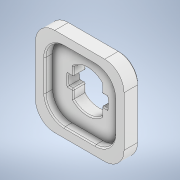
# Autodesk Inventor part: Capinsert_front
Saved by Autodesk Inventor 2021 (Build 250183000, 183)
## iProperties
Created: 2022-04-22
Part Number: Capinsert_front
Material: PPS-Kunststoff
Document SubType Name: Modeling
Designer: Timo
Density: 1.637 g/cm^3
Appearance: Glatt - Weiß
Mass: 2.02617 g
Surface Area: 14.372 cm^2
Volume: 1.23774 cm^3
Author: Timo
Autodesk Inventor part; units mm, degrees
ref_plane "YZ Plane" through (0, 0, 0) normal (1, 0, 0) x (0, 1, 0)
ref_plane "XZ Plane" through (0, 0, 0) normal (0, 1, 0) x (-1, 0, 0)
ref_plane "XY Plane" through (0, 0, 0) normal (0, 0, 1) x (1, 0, 0)
sketch "Skizze1" plane through (0, 0, 0) normal (0, 0, 1) x (1, 0, 0)
  line L0 (-11.45, -11.45) -> (11.45, -11.45)
  line L1 (11.45, -11.45) -> (11.45, 11.45)
  line L2 (11.45, 11.45) -> (-11.45, 11.45)
  line L3 (-11.45, 11.45) -> (-11.45, -11.45)
  line L4 (-11.45, -11.45) -> (11.45, 11.45) construction
  line L5 (11.45, -11.45) -> (-11.45, 11.45) construction
  point P0 (0, 0)
  dimension "d0" = 22.9
  constraints: 12 end point, 2 midpoint, 2 parallel, 2 perpendicular, 1 horizontal
  measures "d0" distance of L2.end L1.end
extrude "Extrusion1" add sketch "Skizze1" along normal blind 3.8
fillet "Rundung1" radius 5 4 edges at (11.45, 11.45, 1.9) (11.45, -11.45, 1.9) (-11.45, -11.45, 1.9) (-11.45, 11.45, 1.9)
sketch "Skizze2" plane through (0, 0, 3.8) normal (0, 0, 1) x (1, 0, 0)
  line L0 (-9, -9) -> (9, -9)
  line L1 (9, -9) -> (9, 9)
  line L2 (9, 9) -> (-9, 9)
  line L3 (-9, 9) -> (-9, -9)
  line L4 (-9, -9) -> (9, 9) construction
  line L5 (9, -9) -> (-9, 9) construction
  point P0 (0, 0)
  dimension "d5" = 18
  dimension "d6" = 18
  constraints: 12 end point, 2 midpoint, 2 parallel, 1 horizontal, 1 perpendicular
  measures "d5" distance of L2.end L1.end
  measures "d6" distance of L1.end L0.end
extrude "Extrusion2" cut sketch "Skizze2" against normal blind 2
fillet "Rundung2" radius 5 4 edges at (-9, 9, 2.8) (9, 9, 2.8) (-9, -9, 2.8) (9, -9, 2.8)
sketch "Skizze3" plane through (0, 0, 1.8) normal (0, 0, 1) x (1, 0, 0)
  circle A0 centre (0, 0) radius 5.2
  line L0 (-3.7, -3.6538) -> (3.7, -3.6538) construction
  line L1 (3.7, -3.6538) -> (3.7, 3.6538)
  line L2 (3.7, 3.6538) -> (-3.7, 3.6538) construction
  line L3 (-3.7, 3.6538) -> (-3.7, -3.6538)
  line L4 (-3.7, -3.6538) -> (3.7, 3.6538) construction
  line L5 (3.7, -3.6538) -> (-3.7, 3.6538) construction
  point P0 (-3.7, 3.6538)
  point P1 (-3.7, -3.6538)
  point P2 (3.7, -3.6538)
  dimension "d10" = 10.4
  dimension "d11" = 7.4
  constraints: 12 end point, 2 midpoint, 2 parallel, 1 coincident, 1 horizontal, 1 perpendicular, 3 other
  measures "d11" distance of L2.end L1.end
extrude "Extrusion3" cut sketch "Skizze3" against normal through all contours L1 A0 L3
sketch "Skizze4" plane through (0, 0, 1.8) normal (0, 0, 1) x (1, 0, 0)
  arc A0 (3.7, 3.6538) -> (-3.7, 3.6538) centre (0, 0) ccw construction
  arc A1 (-3.7, -3.6538) -> (3.7, -3.6538) centre (0, 0) ccw construction
  line L0 (-3.7, -3.6538) -> (-3.7, 3.6538) projected
  line L1 (3.7, 3.6538) -> (3.7, -3.6538) projected
  circle A2 centre (0, 0) radius 5.2
  line L2 (-5.2, -1.35) -> (5.2, -1.35)
  line L3 (5.2, -1.35) -> (5.2, 1.35)
  line L4 (5.2, 1.35) -> (-5.2, 1.35)
  line L5 (-5.2, 1.35) -> (-5.2, -1.35)
  line L6 (-5.2, -1.35) -> (5.2, 1.35) construction
  line L7 (5.2, -1.35) -> (-5.2, 1.35) construction
  point P0 (5.2, 0)
  point P1 (3.7, 1.35)
  point P2 (3.7, -1.35)
  point P3 (-3.7, -1.35)
  point P4 (-3.7, 1.35)
  point P5 (5.0217, 1.35)
  point P6 (5.0217, -1.35)
  point P7 (-5.0217, 1.35)
  point P8 (-5.0217, -1.35)
  dimension "d14" = 2.7
  constraints: 12 end point, 3 midpoint, 2 parallel, 1 coincident, 1 horizontal, 1 perpendicular, 4 other
  measures "d14" distance of L2.end L3.end
extrude "Extrusion4" cut sketch "Skizze4" against normal through all contours L2 A2 L4 L0 | L1 L4 A2 L2
sketch "Skizze5" plane through (0, 0, 0) normal (0, 0, -1) x (-1, 0, 0)
  arc A0 (11.45, 6.45) -> (6.45, 11.45) centre (6.45, 6.45) ccw projected
  line L0 (-6.45, 11.45) -> (6.45, 11.45) projected
  arc A1 (-6.45, 11.45) -> (-11.45, 6.45) centre (-6.45, 6.45) ccw projected
  line L1 (-11.45, -6.45) -> (-11.45, 6.45) projected
  arc A2 (-11.45, -6.45) -> (-6.45, -11.45) centre (-6.45, -6.45) ccw projected
  line L2 (6.45, -11.45) -> (-6.45, -11.45) projected
  arc A3 (6.45, -11.45) -> (11.45, -6.45) centre (6.45, -6.45) ccw projected
  line L3 (11.45, 6.45) -> (11.45, -6.45) projected
  line L4 (-3.7, -1.35) -> (-5.0217, -1.35) projected
  arc A4 (-5.0217, 1.35) -> (-5.0217, -1.35) centre (0, 0) ccw projected
  line L5 (-5.0217, 1.35) -> (-3.7, 1.35) projected
  line L6 (-3.7, 1.35) -> (-3.7, 3.6538) projected
  arc A5 (3.7, 3.6538) -> (-3.7, 3.6538) centre (0, 0) ccw projected
  line L7 (3.7, 3.6538) -> (3.7, 1.35) projected
  line L8 (3.7, 1.35) -> (5.0217, 1.35) projected
  arc A6 (5.0217, -1.35) -> (5.0217, 1.35) centre (0, 0) ccw projected
  line L9 (5.0217, -1.35) -> (3.7, -1.35) projected
  line L10 (3.7, -1.35) -> (3.7, -3.6538) projected
  arc A7 (-3.7, -3.6538) -> (3.7, -3.6538) centre (0, 0) ccw projected
  line L11 (-3.7, -3.6538) -> (-3.7, -1.35) projected
  circle A8 centre (0, 0) radius 6.45
  dimension "d17" = 12.9
  constraints: 1 centre point, 1 coincident
  measures "d17" diameter of A8
extrude "Extrusion5" add sketch "Skizze5" along normal blind 1.5 contours A8
chamfer "Fase1" distance 0.3 angle 45 8 edges at (0, 9, 3.8) (7.5355, 7.5355, 3.8) (9, 0, 3.8) (7.5355, -7.5355, 3.8) (0, -9, 3.8) (-7.5355, -7.5355, 3.8) (-9, 0, 3.8) (-7.5355, 7.5355, 3.8)
chamfer "Fase2" distance 0.3 angle 45 8 edges at (11.45, 0, 0) (9.9855, 9.9855, 0) (0, 11.45, 0) (-9.9855, 9.9855, 0) (-11.45, 0, 0) (-9.9855, -9.9855, 0) (0, -11.45, 0) (9.9855, -9.9855, 0)
fillet "Rundung3" radius 0.3 12 edges at (3.7, -2.5019, -1.5) (0, -5.2, -1.5) (-3.7, -2.5019, -1.5) (-4.3609, -1.35, -1.5) (-5.2, 0, -1.5) (-4.3609, 1.35, -1.5) (-3.7, 2.5019, -1.5) (0, 5.2, -1.5) (3.7, 2.5019, -1.5) (4.3609, 1.35, -1.5) (5.2, 0, -1.5) (4.3609, -1.35, -1.5)
fillet "Rundung4" radius 0.3 12 edges at (0, -5.2, 1.8) (0, 5.2, 1.8) (3.7, -2.5019, 1.8) (4.3609, -1.35, 1.8) (5.2, 0, 1.8) (-5.2, 0, 1.8) (4.3609, 1.35, 1.8) (3.7, 2.5019, 1.8) (-3.7, 2.5019, 1.8) (-4.3609, 1.35, 1.8) (-4.3609, -1.35, 1.8) (-3.7, -2.5019, 1.8)
fillet "Rundung5" radius 0.3 12 edges at (-3.7, 1.35, 0.15) (-3.7879, 1.4379, -1.4121) (-3.7878, 1.4378, 1.7122) (-3.7878, -1.4378, 1.7122) (-3.7879, -1.4379, -1.4121) (-3.7, -1.35, 0.15) (3.7879, -1.4379, -1.4121) (3.7878, -1.4378, 1.7122) (3.7, -1.35, 0.15) (3.7878, 1.4378, 1.7122) (3.7879, 1.4379, -1.4121) (3.7, 1.35, 0.15)
